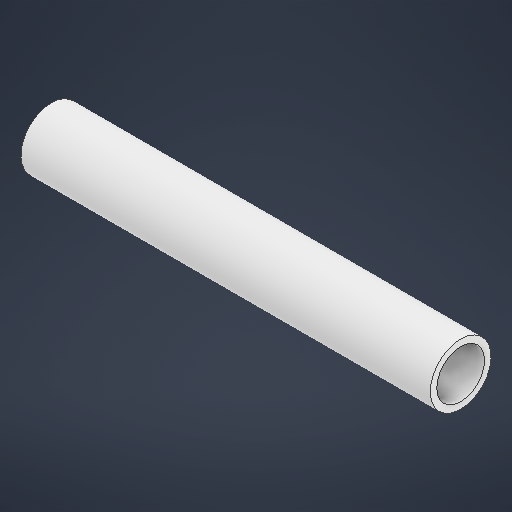
# Autodesk Inventor part: Horizontal Pipe
Saved by Autodesk Inventor 2027 (Build 310192000, 192)
## iProperties
Created: 2026-04-30
Part Number: Horizontal Pipe
Material: PVC-Piping
Document SubType Name: Modeling
Designer: bhoga
Density: 1.4 g/cm^3
Appearance: Smooth - White
Author: bhoga
Autodesk Inventor part; units mm, degrees
ref_plane "YZ Plane" through (0, 0, 0) normal (1, 0, 0) x (0, 1, 0)
ref_plane "XZ Plane" through (0, 0, 0) normal (0, 1, 0) x (-1, 0, 0)
ref_plane "XY Plane" through (0, 0, 0) normal (0, 0, 1) x (1, 0, 0)
sketch "Sketch1" plane through (0, 0, 0) normal (1, 0, 0) x (0, 1, 0)
  circle A0 centre (0, 0) radius 11.15
  circle A1 centre (0, 0) radius 8.755
  dimension "d0" = 22.3
  dimension "d1" = 17.51
  constraints: 2 centre point, 2 coincident
  measures "d0" diameter of A0
  measures "d1" diameter of A1
extrude "Extrusion1" add sketch "Sketch1" along normal blind 150
body "Solid1"
